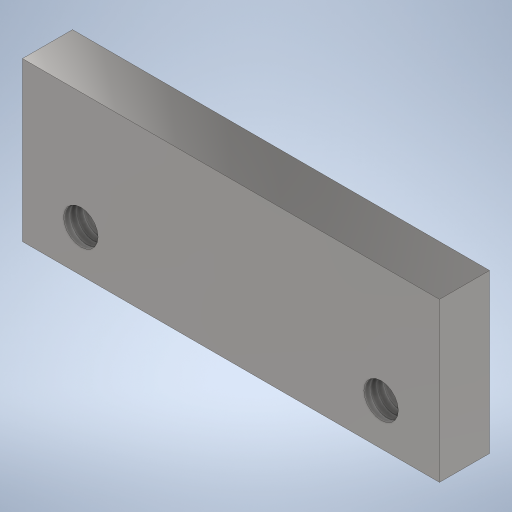
# Autodesk Inventor part: Funrungesch
Saved by Autodesk Inventor 2023.2 (Build 272271000, 271)
## iProperties
Created: 2023-02-02
Part Number: Funrungesch
Material: Steel, Mild
Document SubType Name: Modeling
Designer: Aditya
Density: 7.85 g/cm^3
Appearance: Semi-Polished
Author: Aditya
Autodesk Inventor part; units mm, degrees
ref_plane "YZ Plane" through (0, 0, 0) normal (1, 0, 0) x (0, 1, 0)
ref_plane "XZ Plane" through (0, 0, 0) normal (0, 1, 0) x (-1, 0, 0)
ref_plane "XY Plane" through (0, 0, 0) normal (0, 0, 1) x (1, 0, 0)
sketch "Sketch1" plane through (0, 0, 0) normal (0, 0, 1) x (1, 0, 0)
  line L0 (-25, -9.5) -> (25, -9.5)
  line L1 (25, -9.5) -> (25, 9.5)
  line L2 (25, 9.5) -> (-25, 9.5)
  line L3 (-25, 9.5) -> (-25, -9.5)
  line L4 (-25, -9.5) -> (25, 9.5) construction
  line L5 (25, -9.5) -> (-25, 9.5) construction
  point P0 (0, 0)
  dimension "d0" = 50
  dimension "d1" = 19
  constraints: 12 end point, 2 midpoint, 2 parallel, 1 horizontal, 1 perpendicular
  measures "d0" distance of L2.end L1.end
  measures "d1" distance of L1.end L0.end
extrude "Extrusion1" add sketch "Sketch1" along normal blind 6
sketch "Sketch2" plane through (0, 0, 6) normal (0, 0, 1) x (1, 0, 0)
  line L0 (-25, -9.5) -> (25, -9.5) projected
  line L1 (-25, 9.5) -> (-25, -9.5) projected
  line L2 (25, -9.5) -> (25, 9.5) projected
  point P0 (0, 0)
  point P1 (-18, -4.5)
  point P2 (18, -4.5)
  dimension "d4" = 5
  dimension "d5" = 5
  dimension "d6" = 7
  dimension "d7" = 7
  measures "d4" distance from line of L0 point (-18, -4.5)
  measures "d5" distance from line of L0 point (18, -4.5)
  measures "d6" distance from line of L1 point (-18, -4.5)
  measures "d7" distance from line of L2 point (18, -4.5)
hole "Hole1" at (-18, -4.5, 6) at (18, -4.5, 6) direction (0, 0, -1) diameter 4.134 depth 6 thread size "M5x0.8" class "6H" standard "ISO Metric profile"
body "Solid1"
